Autodesk Fusion 360 part; units mm, degrees
note: some values were not read from the file. Set by a fixed rule: which face or edge a step refers to.
(part 7 of 20)
  spline S38 degree 5 poles (-7.9771, -12.1359) (-7.9772, -12.1359) (-7.9772, -12.136) (-7.9774, -12.1362) (-7.9776, -12.1365) (-7.9779, -12.137) (-7.9782, -12.1375) (-7.9786, -12.1381) (-7.979, -12.1388) (-7.9794, -12.1395) (-7.9799, -12.1403) (-7.9804, -12.1411) (-7.981, -12.1421) (-7.9816, -12.1431) (-7.9823, -12.1441) (-7.9829, -12.1452) (-7.9836, -12.1464) (-7.9844, -12.1477) (-7.9852, -12.149) (-7.986, -12.1504) (-7.9868, -12.1518) (-7.9877, -12.1533) (-7.9886, -12.1549) (-7.9896, -12.1565) (-7.9905, -12.1582) (-7.9915, -12.16) (-7.9926, -12.1618) (-7.9936, -12.1637) (-7.9947, -12.1656) (-7.9958, -12.1676) (-7.997, -12.1696) (-7.9982, -12.1718) (-7.9994, -12.1739) (-8.0006, -12.1762) (-8.0018, -12.1785) (-8.0031, -12.1808) (-8.0044, -12.1832) (-8.0057, -12.1857) (-8.0071, -12.1882) (-8.0084, -12.1908) (-8.0098, -12.1934) (-8.0113, -12.1961) (-8.0127, -12.1988) (-8.0142, -12.2016) (-8.0156, -12.2045) (-8.0171, -12.2074) (-8.0187, -12.2104) (-8.0202, -12.2134) (-8.0218, -12.2164) (-8.0233, -12.2196) (-8.0249, -12.2228) (-8.0265, -12.226) (-8.0282, -12.2293) (-8.0298, -12.2326) (-8.0315, -12.236) (-8.0332, -12.2395) (-8.0349, -12.243) (-8.0366, -12.2465) (-8.0383, -12.2501) (-8.0401, -12.2538) (-8.0419, -12.2575) (-8.0436, -12.2612) (-8.0454, -12.265) (-8.0472, -12.2689) (-8.0491, -12.2728) (-8.0509, -12.2768) (-8.0527, -12.2808) (-8.0546, -12.2848) (-8.0565, -12.289) (-8.0584, -12.2931) (-8.0603, -12.2973) (-8.0622, -12.3016) (-8.0641, -12.3059) (-8.066, -12.3102) (-8.068, -12.3146) (-8.0699, -12.3191) (-8.0719, -12.3236) (-8.0739, -12.3281) (-8.0759, -12.3327) (-8.0779, -12.3374) (-8.0799, -12.3421) (-8.0819, -12.3468) (-8.0839, -12.3516) (-8.0859, -12.3564) (-8.088, -12.3613) (-8.09, -12.3662) (-8.0921, -12.3712) (-8.0941, -12.3762) (-8.0962, -12.3813) (-8.0983, -12.3864) (-8.1004, -12.3915) (-8.1025, -12.3967) (-8.1046, -12.402) (-8.1067, -12.4073) (-8.1088, -12.4126) (-8.1109, -12.418) (-8.113, -12.4234) (-8.1151, -12.4289) (-8.1173, -12.4344) (-8.1194, -12.4399) (-8.1215, -12.4455) (-8.1237, -12.4512) (-8.1258, -12.4568) (-8.128, -12.4626) (-8.1302, -12.4683) (-8.1323, -12.4742) (-8.1345, -12.48) (-8.1366, -12.4859) (-8.1388, -12.4919) (-8.141, -12.4979) (-8.1432, -12.5039) (-8.1453, -12.51) (-8.1475, -12.5161) (-8.1497, -12.5222) (-8.1519, -12.5284) (-8.1541, -12.5347) (-8.1563, -12.5409) (-8.1584, -12.5473) (-8.1606, -12.5536) (-8.1628, -12.56) (-8.165, -12.5665) (-8.1672, -12.5729) (-8.1694, -12.5795) (-8.1716, -12.586) (-8.1738, -12.5926) (-8.176, -12.5993) (-8.1782, -12.606) (-8.1803, -12.6127) (-8.1825, -12.6195) (-8.1847, -12.6263) (-8.1869, -12.6331) (-8.1891, -12.64) (-8.1913, -12.6469) (-8.1935, -12.6539) (-8.1956, -12.6609) (-8.1978, -12.6679) (-8.2, -12.675) (-8.2022, -12.6821) (-8.2044, -12.6893) (-8.2065, -12.6965) (-8.2087, -12.7037) (-8.2109, -12.711) (-8.213, -12.7183) (-8.2152, -12.7256) (-8.2173, -12.733) (-8.2195, -12.7404) (-8.2216, -12.7479) (-8.2238, -12.7554) (-8.2259, -12.7629) (-8.2281, -12.7705) (-8.2302, -12.7781) (-8.2323, -12.7857) (-8.2345, -12.7934) (-8.2366, -12.8011) (-8.2387, -12.8089) (-8.2408, -12.8167) (-8.2429, -12.8245) (-8.245, -12.8324) (-8.2471, -12.8403) (-8.2492, -12.8482) (-8.2513, -12.8562) (-8.2534, -12.8642) (-8.2554, -12.8722) (-8.2575, -12.8803) (-8.2596, -12.8884) (-8.2616, -12.8966) (-8.2637, -12.9048) (-8.2657, -12.913) (-8.2678, -12.9212) (-8.2698, -12.9295) (-8.2718, -12.9379) (-8.2738, -12.9462) (-8.2759, -12.9546) (-8.2779, -12.963) (-8.2799, -12.9715) (-8.2818, -12.98) (-8.2838, -12.9885) (-8.2858, -12.9971) (-8.2878, -13.0057) (-8.2897, -13.0143) (-8.2917, -13.023) (-8.2936, -13.0317) (-8.2956, -13.0404) (-8.2975, -13.0492) (-8.2994, -13.058) (-8.3013, -13.0668) (-8.3032, -13.0757) (-8.3051, -13.0846) (-8.307, -13.0935) (-8.3089, -13.1025) (-8.3107, -13.1115) (-8.3126, -13.1205) (-8.3145, -13.1296) (-8.3163, -13.1386) (-8.3181, -13.1478) (-8.3199, -13.1569) (-8.3218, -13.1661) (-8.3236, -13.1753) (-8.3254, -13.1846) (-8.3271, -13.1939) (-8.3289, -13.2032) (-8.3307, -13.2125) (-8.3324, -13.2219) (-8.3342, -13.2313) (-8.3359, -13.2408) (-8.3376, -13.2503) (-8.3393, -13.2598) (-8.341, -13.2693) (-8.3427, -13.2789) (-8.3444, -13.2885) (-8.3461, -13.2981) (-8.3477, -13.3078) (-8.3494, -13.3174) (-8.351, -13.3272) (-8.3526, -13.3369) (-8.3542, -13.3467) (-8.3558, -13.3565) (-8.3574, -13.3663) (-8.359, -13.3762) (-8.3606, -13.3861) (-8.3621, -13.396) (-8.3637, -13.406) (-8.3652, -13.416) (-8.3667, -13.426) (-8.3682, -13.4361) (-8.3697, -13.4461) (-8.3712, -13.4563) (-8.3726, -13.4664) (-8.3741, -13.4766) (-8.3755, -13.4867) (-8.377, -13.497) (-8.3784, -13.5072) (-8.3798, -13.5175) (-8.3812, -13.5278) (-8.3826, -13.5382) (-8.3839, -13.5485) (-8.3853, -13.5589) (-8.3866, -13.5693) (-8.3879, -13.5798) (-8.3893, -13.5903) (-8.3906, -13.6008) (-8.3916, -13.6092) (-8.3924, -13.6155) (-8.3929, -13.6198) (-8.3931, -13.6219) knots 0 0 0 0 0 0 0.00416667 0.00833333 0.0125 0.01666667 0.02083333 0.025 0.02916667 0.03333333 0.0375 0.04166667 0.04583333 0.05 0.05416667 0.05833333 0.0625 0.06666667 0.07083333 0.075 0.07916667 0.08333333 0.0875 0.09166667 0.09583333 0.1 0.10416667 0.10833333 0.1125 0.11666667 0.12083333 0.125 0.12916667 0.13333333 0.1375 0.14166667 0.14583333 0.15 0.15416667 0.15833333 0.1625 0.16666667 0.17083333 0.175 0.17916667 0.18333333 0.1875 0.19166667 0.19583333 0.2 0.20416667 0.20833333 0.2125 0.21666667 0.22083333 0.225 0.22916667 0.23333333 0.2375 0.24166667 0.24583333 0.25 0.25416667 0.25833333 0.2625 0.26666667 0.27083333 0.275 0.27916667 0.28333333 0.2875 0.29166667 0.29583333 0.3 0.30416667 0.30833333 0.3125 0.31666667 0.32083333 0.325 0.32916667 0.33333333 0.3375 0.34166667 0.34583333 0.35 0.35416667 0.35833333 0.3625 0.36666667 0.37083333 0.375 0.37916667 0.38333333 0.3875 0.39166667 0.39583333 0.4 0.40416667 0.40833333 0.4125 0.41666667 0.42083333 0.425 0.42916667 0.43333333 0.4375 0.44166667 0.44583333 0.45 0.45416667 0.45833333 0.4625 0.46666667 0.47083333 0.475 0.47916667 0.48333333 0.4875 0.49166667 0.49583333 0.5 0.50416667 0.50833333 0.5125 0.51666667 0.52083333 0.525 0.52916667 0.53333333 0.5375 0.54166667 0.54583333 0.55 0.55416667 0.55833333 0.5625 0.56666667 0.57083333 0.575 0.57916667 0.58333333 0.5875 0.59166667 0.59583333 0.6 0.60416667 0.60833333 0.6125 0.61666667 0.62083333 0.625 0.62916667 0.63333333 0.6375 0.64166667 0.64583333 0.65 0.65416667 0.65833333 0.6625 0.66666667 0.67083333 0.675 0.67916667 0.68333333 0.6875 0.69166667 0.69583333 0.7 0.70416667 0.70833333 0.7125 0.71666667 0.72083333 0.725 0.72916667 0.73333333 0.7375 0.74166667 0.74583333 0.75 0.75416667 0.75833333 0.7625 0.76666667 0.77083333 0.775 0.77916667 0.78333333 0.7875 0.79166667 0.79583333 0.8 0.80416667 0.80833333 0.8125 0.81666667 0.82083333 0.825 0.82916667 0.83333333 0.8375 0.84166667 0.84583333 0.85 0.85416667 0.85833333 0.8625 0.86666667 0.87083333 0.875 0.87916667 0.88333333 0.8875 0.89166667 0.89583333 0.9 0.90416667 0.90833333 0.9125 0.91666667 0.92083333 0.925 0.92916667 0.93333333 0.9375 0.94166667 0.94583333 0.95 0.95416667 0.95833333 0.9625 0.96666667 0.97083333 0.975 0.97916667 0.98333333 0.9875 0.99166667 0.99583333 1 1 1 1 1 1
  spline S39 degree 5 poles (-7.6003, -14.0796) (-7.5986, -14.0783) (-7.5952, -14.0758) (-7.5901, -14.0719) (-7.5833, -14.0668) (-7.5749, -14.0604) (-7.5665, -14.0541) (-7.5581, -14.0477) (-7.5497, -14.0413) (-7.5414, -14.035) (-7.5331, -14.0286) (-7.5248, -14.0222) (-7.5166, -14.0159) (-7.5084, -14.0095) (-7.5002, -14.0032) (-7.4921, -13.9968) (-7.484, -13.9905) (-7.4759, -13.9841) (-7.4679, -13.9778) (-7.4599, -13.9714) (-7.4519, -13.9651) (-7.4439, -13.9588) (-7.436, -13.9525) (-7.4281, -13.9461) (-7.4203, -13.9398) (-7.4124, -13.9335) (-7.4046, -13.9272) (-7.3969, -13.9209) (-7.3892, -13.9146) (-7.3815, -13.9083) (-7.3738, -13.902) (-7.3662, -13.8958) (-7.3586, -13.8895) (-7.351, -13.8832) (-7.3435, -13.8769) (-7.336, -13.8707) (-7.3285, -13.8644) (-7.321, -13.8582) (-7.3136, -13.8519) (-7.3063, -13.8457) (-7.2989, -13.8395) (-7.2916, -13.8333) (-7.2843, -13.827) (-7.2771, -13.8208) (-7.2699, -13.8146) (-7.2627, -13.8084) (-7.2555, -13.8023) (-7.2484, -13.7961) (-7.2413, -13.7899) (-7.2343, -13.7837) (-7.2272, -13.7776) (-7.2203, -13.7714) (-7.2133, -13.7653) (-7.2064, -13.7592) (-7.1995, -13.753) (-7.1926, -13.7469) (-7.1858, -13.7408) (-7.179, -13.7347) (-7.1723, -13.7286) (-7.1655, -13.7226) (-7.1588, -13.7165) (-7.1522, -13.7104) (-7.1455, -13.7044) (-7.1389, -13.6983) (-7.1324, -13.6923) (-7.1259, -13.6863) (-7.1194, -13.6803) (-7.1129, -13.6743) (-7.1065, -13.6683) (-7.1001, -13.6623) (-7.0937, -13.6563) (-7.0874, -13.6504) (-7.0811, -13.6444) (-7.0748, -13.6385) (-7.0686, -13.6325) (-7.0624, -13.6266) (-7.0562, -13.6207) (-7.0501, -13.6148) (-7.044, -13.6089) (-7.0379, -13.6031) (-7.0319, -13.5972) (-7.0259, -13.5914) (-7.02, -13.5855) (-7.014, -13.5797) (-7.0081, -13.5739) (-7.0023, -13.5681) (-6.9965, -13.5624) (-6.9907, -13.5566) (-6.9849, -13.5508) (-6.9792, -13.5451) (-6.9735, -13.5394) (-6.9678, -13.5337) (-6.9622, -13.528) (-6.9566, -13.5223) (-6.9511, -13.5166) (-6.9455, -13.511) (-6.94, -13.5053) (-6.9346, -13.4997) (-6.9292, -13.4941) (-6.9238, -13.4885) (-6.9184, -13.4829) (-6.9131, -13.4774) (-6.9078, -13.4718) (-6.9026, -13.4663) (-6.8974, -13.4608) (-6.8922, -13.4553) (-6.8871, -13.4498) (-6.8819, -13.4444) (-6.8769, -13.4389) (-6.8718, -13.4335) (-6.8668, -13.4281) (-6.8618, -13.4227) (-6.8569, -13.4173) (-6.852, -13.412) (-6.8471, -13.4066) (-6.8423, -13.4013) (-6.8375, -13.396) (-6.8327, -13.3907) (-6.828, -13.3855) (-6.8233, -13.3802) (-6.8187, -13.375) (-6.814, -13.3698) (-6.8094, -13.3646) (-6.8049, -13.3595) (-6.8004, -13.3543) (-6.7959, -13.3492) (-6.7914, -13.3441) (-6.787, -13.339) (-6.7826, -13.334) (-6.7783, -13.329) (-6.774, -13.3239) (-6.7697, -13.319) (-6.7655, -13.314) (-6.7613, -13.309) (-6.7571, -13.3041) (-6.753, -13.2992) (-6.7489, -13.2944) (-6.7448, -13.2895) (-6.7408, -13.2847) (-6.7368, -13.2799) (-6.7328, -13.2751) (-6.7289, -13.2703) (-6.725, -13.2656) (-6.7212, -13.2609) (-6.7174, -13.2562) (-6.7136, -13.2516) (-6.7098, -13.2469) (-6.7061, -13.2423) (-6.7025, -13.2378) (-6.6988, -13.2332) (-6.6952, -13.2287) (-6.6917, -13.2242) (-6.6881, -13.2197) (-6.6846, -13.2153) (-6.6812, -13.2109) (-6.6778, -13.2065) (-6.6744, -13.2022) (-6.671, -13.1978) (-6.6677, -13.1935) (-6.6644, -13.1893) (-6.6612, -13.185) (-6.658, -13.1808) (-6.6548, -13.1767) (-6.6517, -13.1725) (-6.6486, -13.1684) (-6.6455, -13.1643) (-6.6425, -13.1603) (-6.6395, -13.1563) (-6.6366, -13.1523) (-6.6337, -13.1483) (-6.6308, -13.1444) (-6.628, -13.1405) (-6.6252, -13.1367) (-6.6224, -13.1328) (-6.6197, -13.1291) (-6.617, -13.1253) (-6.6143, -13.1216) (-6.6117, -13.1179) (-6.6091, -13.1143) (-6.6065, -13.1107) (-6.604, -13.1071) (-6.6016, -13.1036) (-6.5991, -13.1001) (-6.5967, -13.0966) (-6.5944, -13.0932) (-6.592, -13.0898) (-6.5897, -13.0865) (-6.5875, -13.0832) (-6.5853, -13.0799) (-6.5831, -13.0767) (-6.581, -13.0735) (-6.5788, -13.0703) (-6.5768, -13.0672) (-6.5747, -13.0642) (-6.5728, -13.0612) (-6.5708, -13.0582) (-6.5689, -13.0553) (-6.567, -13.0524) (-6.5651, -13.0495) (-6.5633, -13.0467) (-6.5616, -13.044) (-6.5598, -13.0413) (-6.5581, -13.0386) (-6.5565, -13.036) (-6.5549, -13.0334) (-6.5533, -13.0309) (-6.5517, -13.0284) (-6.5502, -13.026) (-6.5488, -13.0236) (-6.5473, -13.0213) (-6.5459, -13.019) (-6.5446, -13.0168) (-6.5433, -13.0146) (-6.542, -13.0125) (-6.5407, -13.0104) (-6.5395, -13.0084) (-6.5384, -13.0064) (-6.5372, -13.0045) (-6.5361, -13.0027) (-6.5351, -13.0009) (-6.5341, -12.9991) (-6.5331, -12.9974) (-6.5321, -12.9958) (-6.5312, -12.9942) (-6.5304, -12.9927) (-6.5295, -12.9913) (-6.5288, -12.9899) (-6.528, -12.9885) (-6.5273, -12.9873) (-6.5266, -12.986) (-6.526, -12.9849) (-6.5254, -12.9838) (-6.5248, -12.9828) (-6.5243, -12.9818) (-6.5238, -12.9809) (-6.5234, -12.9801) (-6.523, -12.9794) (-6.5226, -12.9787) (-6.5223, -12.9781) (-6.522, -12.9775) (-6.5218, -12.977) (-6.5216, -12.9767) (-6.5215, -12.9765) (-6.5214, -12.9764) (-6.5214, -12.9763) knots -1 -1 -1 -1 -1 -1 -0.99583333 -0.99166667 -0.9875 -0.98333333 -0.97916667 -0.975 -0.97083333 -0.96666667 -0.9625 -0.95833333 -0.95416667 -0.95 -0.94583333 -0.94166667 -0.9375 -0.93333333 -0.92916667 -0.925 -0.92083333 -0.91666667 -0.9125 -0.90833333 -0.90416667 -0.9 -0.89583333 -0.89166667 -0.8875 -0.88333333 -0.87916667 -0.875 -0.87083333 -0.86666667 -0.8625 -0.85833333 -0.85416667 -0.85 -0.84583333 -0.84166667 -0.8375 -0.83333333 -0.82916667 -0.825 -0.82083333 -0.81666667 -0.8125 -0.80833333 -0.80416667 -0.8 -0.79583333 -0.79166667 -0.7875 -0.78333333 -0.77916667 -0.775 -0.77083333 -0.76666667 -0.7625 -0.75833333 -0.75416667 -0.75 -0.74583333 -0.74166667 -0.7375 -0.73333333 -0.72916667 -0.725 -0.72083333 -0.71666667 -0.7125 -0.70833333 -0.70416667 -0.7 -0.69583333 -0.69166667 -0.6875 -0.68333333 -0.67916667 -0.675 -0.67083333 -0.66666667 -0.6625 -0.65833333 -0.65416667 -0.65 -0.64583333 -0.64166667 -0.6375 -0.63333333 -0.62916667 -0.625 -0.62083333 -0.61666667 -0.6125 -0.60833333 -0.60416667 -0.6 -0.59583333 -0.59166667 -0.5875 -0.58333333 -0.57916667 -0.575 -0.57083333 -0.56666667 -0.5625 -0.55833333 -0.55416667 -0.55 -0.54583333 -0.54166667 -0.5375 -0.53333333 -0.52916667 -0.525 -0.52083333 -0.51666667 -0.5125 -0.50833333 -0.50416667 -0.5 -0.49583333 -0.49166667 -0.4875 -0.48333333 -0.47916667 -0.475 -0.47083333 -0.46666667 -0.4625 -0.45833333 -0.45416667 -0.45 -0.44583333 -0.44166667 -0.4375 -0.43333333 -0.42916667 -0.425 -0.42083333 -0.41666667 -0.4125 -0.40833333 -0.40416667 -0.4 -0.39583333 -0.39166667 -0.3875 -0.38333333 -0.37916667 -0.375 -0.37083333 -0.36666667 -0.3625 -0.35833333 -0.35416667 -0.35 -0.34583333 -0.34166667 -0.3375 -0.33333333 -0.32916667 -0.325 -0.32083333 -0.31666667 -0.3125 -0.30833333 -0.30416667 -0.3 -0.29583333 -0.29166667 -0.2875 -0.28333333 -0.27916667 -0.275 -0.27083333 -0.26666667 -0.2625 -0.25833333 -0.25416667 -0.25 -0.24583333 -0.24166667 -0.2375 -0.23333333 -0.22916667 -0.225 -0.22083333 -0.21666667 -0.2125 -0.20833333 -0.20416667 -0.2 -0.19583333 -0.19166667 -0.1875 -0.18333333 -0.17916667 -0.175 -0.17083333 -0.16666667 -0.1625 -0.15833333 -0.15416667 -0.15 -0.14583333 -0.14166667 -0.1375 -0.13333333 -0.12916667 -0.125 -0.12083333 -0.11666667 -0.1125 -0.10833333 -0.10416667 -0.1 -0.09583333 -0.09166667 -0.0875 -0.08333333 -0.07916667 -0.075 -0.07083333 -0.06666667 -0.0625 -0.05833333 -0.05416667 -0.05 -0.04583333 -0.04166667 -0.0375 -0.03333333 -0.02916667 -0.025 -0.02083333 -0.01666667 -0.0125 -0.00833333 -0.00416667 0 0 0 0 0 0
  arc A52 (11.0419, 11.5792) -> (10.3616, 12.1917) centre (0, 0) ccw
  line L82 (11.2355, 9.202) -> (11.235, 9.2016)
  spline S40 degree 5 poles (14.4246, 6.9233) (14.4224, 6.9232) (14.4182, 6.9232) (14.4118, 6.9231) (14.4033, 6.9229) (14.3927, 6.9227) (14.3822, 6.9225) (14.3716, 6.9223) (14.3611, 6.9221) (14.3507, 6.9218) (14.3402, 6.9215) (14.3298, 6.9212) (14.3194, 6.9209) (14.309, 6.9206) (14.2987, 6.9203) (14.2883, 6.9199) (14.2781, 6.9195) (14.2678, 6.9192) (14.2576, 6.9188) (14.2474, 6.9183) (14.2372, 6.9179) (14.227, 6.9175) (14.2169, 6.917) (14.2068, 6.9165) (14.1967, 6.916) (14.1867, 6.9155) (14.1767, 6.915) (14.1667, 6.9145) (14.1568, 6.9139) (14.1468, 6.9134) (14.1369, 6.9128) (14.1271, 6.9122) (14.1172, 6.9116) (14.1074, 6.9109) (14.0976, 6.9103) (14.0879, 6.9097) (14.0782, 6.909) (14.0685, 6.9083) (14.0588, 6.9076) (14.0492, 6.9069) (14.0396, 6.9062) (14.03, 6.9055) (14.0205, 6.9047) (14.011, 6.9039) (14.0015, 6.9032) (13.992, 6.9024) (13.9826, 6.9016) (13.9732, 6.9008) (13.9639, 6.8999) (13.9545, 6.8991) (13.9452, 6.8982) (13.936, 6.8974) (13.9267, 6.8965) (13.9175, 6.8956) (13.9083, 6.8947) (13.8992, 6.8938) (13.8901, 6.8929) (13.881, 6.8919) (13.872, 6.891) (13.8629, 6.89) (13.854, 6.889) (13.845, 6.888) (13.8361, 6.887) (13.8272, 6.886) (13.8184, 6.885) (13.8095, 6.884) (13.8007, 6.8829) (13.792, 6.8818) (13.7833, 6.8808) (13.7746, 6.8797) (13.7659, 6.8786) (13.7573, 6.8775) (13.7487, 6.8764) (13.7401, 6.8753) (13.7316, 6.8741) (13.7231, 6.873) (13.7147, 6.8718) (13.7063, 6.8707) (13.6979, 6.8695) (13.6895, 6.8683) (13.6812, 6.8671) (13.6729, 6.8659) (13.6647, 6.8647) (13.6564, 6.8635) (13.6483, 6.8623) (13.6401, 6.861) (13.632, 6.8598) (13.6239, 6.8585) (13.6159, 6.8572) (13.6079, 6.856) (13.5999, 6.8547) (13.592, 6.8534) (13.5841, 6.8521) (13.5762, 6.8508) (13.5684, 6.8494) (13.5606, 6.8481) (13.5528, 6.8468) (13.5451, 6.8454) (13.5375, 6.8441) (13.5298, 6.8427) (13.5222, 6.8414) (13.5146, 6.84) (13.5071, 6.8386) (13.4996, 6.8372) (13.4922, 6.8358) (13.4847, 6.8344) (13.4773, 6.833) (13.47, 6.8316) (13.4627, 6.8302) (13.4554, 6.8288) (13.4482, 6.8273) (13.441, 6.8259) (13.4339, 6.8244) (13.4267, 6.823) (13.4197, 6.8215) (13.4126, 6.8201) (13.4056, 6.8186) (13.3987, 6.8171) (13.3918, 6.8157) (13.3849, 6.8142) (13.378, 6.8127) (13.3712, 6.8112) (13.3645, 6.8097) (13.3578, 6.8082) (13.3511, 6.8067) (13.3445, 6.8052) (13.3379, 6.8037) (13.3313, 6.8022) (13.3248, 6.8007) (13.3183, 6.7992) (13.3119, 6.7976) (13.3055, 6.7961) (13.2991, 6.7946) (13.2928, 6.7931) (13.2866, 6.7915) (13.2804, 6.79) (13.2742, 6.7885) (13.268, 6.7869) (13.2619, 6.7854) (13.2559, 6.7839) (13.2499, 6.7823) (13.2439, 6.7808) (13.238, 6.7792) (13.2321, 6.7777) (13.2263, 6.7761) (13.2205, 6.7746) (13.2147, 6.7731) (13.209, 6.7715) (13.2034, 6.77) (13.1978, 6.7684) (13.1922, 6.7669) (13.1867, 6.7653) (13.1812, 6.7638) (13.1758, 6.7623) (13.1704, 6.7607) (13.165, 6.7592) (13.1597, 6.7577) (13.1545, 6.7561) (13.1493, 6.7546) (13.1441, 6.7531) (13.139, 6.7516) (13.1339, 6.75) (13.1289, 6.7485) (13.124, 6.747) (13.119, 6.7455) (13.1142, 6.744) (13.1093, 6.7425) (13.1046, 6.741) (13.0998, 6.7395) (13.0951, 6.738) (13.0905, 6.7366) (13.0859, 6.7351) (13.0814, 6.7336) (13.0769, 6.7321) (13.0725, 6.7307) (13.0681, 6.7292) (13.0638, 6.7278) (13.0595, 6.7264) (13.0552, 6.7249) (13.0511, 6.7235) (13.0469, 6.7221) (13.0429, 6.7207) (13.0388, 6.7193) (13.0349, 6.7179) (13.0309, 6.7165) (13.0271, 6.7152) (13.0232, 6.7138) (13.0195, 6.7125) (13.0158, 6.7111) (13.0121, 6.7098) (13.0085, 6.7085) (13.005, 6.7072) (13.0015, 6.7059) (12.998, 6.7046) (12.9946, 6.7033) (12.9913, 6.7021) (12.988, 6.7008) (12.9848, 6.6996) (12.9816, 6.6984) (12.9785, 6.6972) (12.9755, 6.696) (12.9725, 6.6948) (12.9695, 6.6937) (12.9667, 6.6925) (12.9638, 6.6914) (12.9611, 6.6903) (12.9584, 6.6892) (12.9557, 6.6881) (12.9531, 6.6871) (12.9506, 6.686) (12.9482, 6.685) (12.9457, 6.684) (12.9434, 6.683) (12.9411, 6.6821) (12.9389, 6.6811) (12.9367, 6.6802) (12.9346, 6.6793) (12.9326, 6.6784) (12.9306, 6.6775) (12.9287, 6.6767) (12.9269, 6.6759) (12.9251, 6.6751) (12.9234, 6.6743) (12.9217, 6.6736) (12.9201, 6.6729) (12.9186, 6.6722) (12.9171, 6.6715) (12.9157, 6.6709) (12.9144, 6.6703) (12.9132, 6.6697) (12.912, 6.6691) (12.9108, 6.6686) (12.9098, 6.6681) (12.9088, 6.6676) (12.9079, 6.6672) (12.9071, 6.6668) (12.9063, 6.6664) (12.9056, 6.6661) (12.905, 6.6658) (12.9044, 6.6655) (12.9039, 6.6652) (12.9036, 6.6651) (12.9034, 6.665) (12.9033, 6.6649) (12.9032, 6.6649) knots -1 -1 -1 -1 -1 -1 -0.99583333 -0.99166667 -0.9875 -0.98333333 -0.97916667 -0.975 -0.97083333 -0.96666667 -0.9625 -0.95833333 -0.95416667 -0.95 -0.94583333 -0.94166667 -0.9375 -0.93333333 -0.92916667 -0.925 -0.92083333 -0.91666667 -0.9125 -0.90833333 -0.90416667 -0.9 -0.89583333 -0.89166667 -0.8875 -0.88333333 -0.87916667 -0.875 -0.87083333 -0.86666667 -0.8625 -0.85833333 -0.85416667 -0.85 -0.84583333 -0.84166667 -0.8375 -0.83333333 -0.82916667 -0.825 -0.82083333 -0.81666667 -0.8125 -0.80833333 -0.80416667 -0.8 -0.79583333 -0.79166667 -0.7875 -0.78333333 -0.77916667 -0.775 -0.77083333 -0.76666667 -0.7625 -0.75833333 -0.75416667 -0.75 -0.74583333 -0.74166667 -0.7375 -0.73333333 -0.72916667 -0.725 -0.72083333 -0.71666667 -0.7125 -0.70833333 -0.70416667 -0.7 -0.69583333 -0.69166667 -0.6875 -0.68333333 -0.67916667 -0.675 -0.67083333 -0.66666667 -0.6625 -0.65833333 -0.65416667 -0.65 -0.64583333 -0.64166667 -0.6375 -0.63333333 -0.62916667 -0.625 -0.62083333 -0.61666667 -0.6125 -0.60833333 -0.60416667 -0.6 -0.59583333 -0.59166667 -0.5875 -0.58333333 -0.57916667 -0.575 -0.57083333 -0.56666667 -0.5625 -0.55833333 -0.55416667 -0.55 -0.54583333 -0.54166667 -0.5375 -0.53333333 -0.52916667 -0.525 -0.52083333 -0.51666667 -0.5125 -0.50833333 -0.50416667 -0.5 -0.49583333 -0.49166667 -0.4875 -0.48333333 -0.47916667 -0.475 -0.47083333 -0.46666667 -0.4625 -0.45833333 -0.45416667 -0.45 -0.44583333 -0.44166667 -0.4375 -0.43333333 -0.42916667 -0.425 -0.42083333 -0.41666667 -0.4125 -0.40833333 -0.40416667 -0.4 -0.39583333 -0.39166667 -0.3875 -0.38333333 -0.37916667 -0.375 -0.37083333 -0.36666667 -0.3625 -0.35833333 -0.35416667 -0.35 -0.34583333 -0.34166667 -0.3375 -0.33333333 -0.32916667 -0.325 -0.32083333 -0.31666667 -0.3125 -0.30833333 -0.30416667 -0.3 -0.29583333 -0.29166667 -0.2875 -0.28333333 -0.27916667 -0.275 -0.27083333 -0.26666667 -0.2625 -0.25833333 -0.25416667 -0.25 -0.24583333 -0.24166667 -0.2375 -0.23333333 -0.22916667 -0.225 -0.22083333 -0.21666667 -0.2125 -0.20833333 -0.20416667 -0.2 -0.19583333 -0.19166667 -0.1875 -0.18333333 -0.17916667 -0.175 -0.17083333 -0.16666667 -0.1625 -0.15833333 -0.15416667 -0.15 -0.14583333 -0.14166667 -0.1375 -0.13333333 -0.12916667 -0.125 -0.12083333 -0.11666667 -0.1125 -0.10833333 -0.10416667 -0.1 -0.09583333 -0.09166667 -0.0875 -0.08333333 -0.07916667 -0.075 -0.07083333 -0.06666667 -0.0625 -0.05833333 -0.05416667 -0.05 -0.04583333 -0.04166667 -0.0375 -0.03333333 -0.02916667 -0.025 -0.02083333 -0.01666667 -0.0125 -0.00833333 -0.00416667 0 0 0 0 0 0
  line L83 (-3.4851, 13.301) -> (-3.6808, 14.048)
  spline S41 degree 5 poles (10.3616, 12.1917) (10.3596, 12.1908) (10.3558, 12.189) (10.35, 12.1863) (10.3423, 12.1828) (10.3327, 12.1783) (10.3231, 12.1738) (10.3136, 12.1693) (10.3041, 12.1648) (10.2946, 12.1603) (10.2852, 12.1558) (10.2758, 12.1513) (10.2664, 12.1468) (10.2571, 12.1423) (10.2478, 12.1378) (10.2385, 12.1332) (10.2292, 12.1287) (10.22, 12.1242) (10.2108, 12.1197) (10.2017, 12.1151) (10.1925, 12.1106) (10.1834, 12.1061) (10.1744, 12.1015) (10.1654, 12.097) (10.1564, 12.0924) (10.1474, 12.0879) (10.1385, 12.0834) (10.1296, 12.0788) (10.1207, 12.0743) (10.1119, 12.0697) (10.1031, 12.0651) (10.0943, 12.0606) (10.0855, 12.056) (10.0768, 12.0515) (10.0682, 12.0469) (10.0595, 12.0423) (10.0509, 12.0378) (10.0423, 12.0332) (10.0338, 12.0287) (10.0253, 12.0241) (10.0168, 12.0195) (10.0084, 12.015) (9.9999, 12.0104) (9.9916, 12.0058) (9.9832, 12.0013) (9.9749, 11.9967) (9.9666, 11.9921) (9.9584, 11.9876) (9.9502, 11.983) (9.942, 11.9785) (9.9338, 11.9739) (9.9257, 11.9693) (9.9176, 11.9648) (9.9096, 11.9602) (9.9016, 11.9557) (9.8936, 11.9511) (9.8857, 11.9465) (9.8777, 11.942) (9.8699, 11.9374) (9.862, 11.9329) (9.8542, 11.9283) (9.8464, 11.9238) (9.8387, 11.9193) (9.831, 11.9147) (9.8233, 11.9102) (9.8157, 11.9056) (9.8081, 11.9011) (9.8005, 11.8966) (9.793, 11.8921) (9.7855, 11.8875) (9.778, 11.883) (9.7706, 11.8785) (9.7632, 11.874) (9.7558, 11.8695) (9.7485, 11.865) (9.7412, 11.8605) (9.7339, 11.856) (9.7267, 11.8515) (9.7195, 11.847) (9.7124, 11.8425) (9.7053, 11.8381) (9.6982, 11.8336) (9.6912, 11.8291) (9.6841, 11.8247) (9.6772, 11.8202) (9.6702, 11.8158) (9.6633, 11.8113) (9.6565, 11.8069) (9.6496, 11.8025) (9.6428, 11.798) (9.6361, 11.7936) (9.6294, 11.7892) (9.6227, 11.7848) (9.616, 11.7804) (9.6094, 11.776) (9.6028, 11.7717) (9.5963, 11.7673) (9.5898, 11.7629) (9.5833, 11.7586) (9.5769, 11.7542) (9.5705, 11.7499) (9.5642, 11.7455) (9.5578, 11.7412) (9.5516, 11.7369) (9.5453, 11.7326) (9.5391, 11.7283) (9.5329, 11.724) (9.5268, 11.7197) (9.5207, 11.7155) (9.5146, 11.7112) (9.5086, 11.707) (9.5026, 11.7027) (9.4967, 11.6985) (9.4908, 11.6943) (9.4849, 11.6901) (9.4791, 11.6859) (9.4733, 11.6817) (9.4675, 11.6775) (9.4618, 11.6733) (9.4561, 11.6692) (9.4505, 11.6651) (9.4449, 11.6609) (9.4393, 11.6568) (9.4338, 11.6527) (9.4283, 11.6486) (9.4228, 11.6446) (9.4174, 11.6405) (9.412, 11.6365) (9.4067, 11.6324) (9.4014, 11.6284) (9.3962, 11.6244) (9.3909, 11.6204) (9.3858, 11.6164) (9.3806, 11.6125) (9.3755, 11.6085) (9.3705, 11.6046) (9.3654, 11.6007) (9.3605, 11.5968) (9.3555, 11.5929) (9.3506, 11.589) (9.3457, 11.5852) (9.3409, 11.5813) (9.3361, 11.5775) (9.3314, 11.5737) (9.3267, 11.5699) (9.322, 11.5662) (9.3174, 11.5624) (9.3128, 11.5587) (9.3083, 11.555) (9.3038, 11.5513) (9.2993, 11.5476) (9.2949, 11.544) (9.2905, 11.5403) (9.2862, 11.5367) (9.2819, 11.5331) (9.2776, 11.5295) (9.2734, 11.526) (9.2692, 11.5224) (9.2651, 11.5189) (9.261, 11.5154) (9.257, 11.512) (9.253, 11.5085) (9.249, 11.5051) (9.2451, 11.5017) (9.2412, 11.4983) (9.2373, 11.495) (9.2335, 11.4916) (9.2298, 11.4883) (9.2261, 11.485) (9.2224, 11.4818) (9.2188, 11.4785) (9.2152, 11.4753) (9.2116, 11.4721) (9.2081, 11.469) (9.2047, 11.4658) (9.2013, 11.4627) (9.1979, 11.4597) (9.1946, 11.4566) (9.1913, 11.4536) (9.188, 11.4506) (9.1848, 11.4476) (9.1817, 11.4447) (9.1786, 11.4418) (9.1755, 11.4389) (9.1725, 11.436) (9.1695, 11.4332) (9.1666, 11.4304) (9.1637, 11.4276) (9.1608, 11.4249) (9.158, 11.4222) (9.1553, 11.4195) (9.1526, 11.4169) (9.1499, 11.4143) (9.1473, 11.4117) (9.1447, 11.4092) (9.1422, 11.4067) (9.1397, 11.4042) (9.1372, 11.4018) (9.1348, 11.3994) (9.1325, 11.397) (9.1302, 11.3947) (9.1279, 11.3924) (9.1257, 11.3902) (9.1235, 11.388) (9.1214, 11.3858) (9.1194, 11.3836) (9.1173, 11.3815) (9.1153, 11.3795) (9.1134, 11.3775) (9.1115, 11.3755) (9.1097, 11.3735) (9.1079, 11.3717) (9.1062, 11.3698) (9.1045, 11.368) (9.1028, 11.3662) (9.1012, 11.3645) (9.0997, 11.3628) (9.0982, 11.3612) (9.0967, 11.3596) (9.0953, 11.3581) (9.0939, 11.3566) (9.0926, 11.3551) (9.0914, 11.3537) (9.0902, 11.3524) (9.089, 11.3511) (9.0879, 11.3498) (9.0868, 11.3486) (9.0858, 11.3475) (9.0849, 11.3464) (9.084, 11.3453) (9.0831, 11.3443) (9.0823, 11.3434) (9.0815, 11.3425) (9.0808, 11.3417) (9.0802, 11.3409) (9.0796, 11.3402) (9.079, 11.3395) (9.0785, 11.3389) (9.0781, 11.3384) (9.0777, 11.3379) (9.0773, 11.3375) (9.0771, 11.3372) (9.0769, 11.337) (9.0769, 11.3369) (9.0768, 11.3369) knots -1 -1 -1 -1 -1 -1 -0.99583333 -0.99166667 -0.9875 -0.98333333 -0.97916667 -0.975 -0.97083333 -0.96666667 -0.9625 -0.95833333 -0.95416667 -0.95 -0.94583333 -0.94166667 -0.9375 -0.93333333 -0.92916667 -0.925 -0.92083333 -0.91666667 -0.9125 -0.90833333 -0.90416667 -0.9 -0.89583333 -0.89166667 -0.8875 -0.88333333 -0.87916667 -0.875 -0.87083333 -0.86666667 -0.8625 -0.85833333 -0.85416667 -0.85 -0.84583333 -0.84166667 -0.8375 -0.83333333 -0.82916667 -0.825 -0.82083333 -0.81666667 -0.8125 -0.80833333 -0.80416667 -0.8 -0.79583333 -0.79166667 -0.7875 -0.78333333 -0.77916667 -0.775 -0.77083333 -0.76666667 -0.7625 -0.75833333 -0.75416667 -0.75 -0.74583333 -0.74166667 -0.7375 -0.73333333 -0.72916667 -0.725 -0.72083333 -0.71666667 -0.7125 -0.70833333 -0.70416667 -0.7 -0.69583333 -0.69166667 -0.6875 -0.68333333 -0.67916667 -0.675 -0.67083333 -0.66666667 -0.6625 -0.65833333 -0.65416667 -0.65 -0.64583333 -0.64166667 -0.6375 -0.63333333 -0.62916667 -0.625 -0.62083333 -0.61666667 -0.6125 -0.60833333 -0.60416667 -0.6 -0.59583333 -0.59166667 -0.5875 -0.58333333 -0.57916667 -0.575 -0.57083333 -0.56666667 -0.5625 -0.55833333 -0.55416667 -0.55 -0.54583333 -0.54166667 -0.5375 -0.53333333 -0.52916667 -0.525 -0.52083333 -0.51666667 -0.5125 -0.50833333 -0.50416667 -0.5 -0.49583333 -0.49166667 -0.4875 -0.48333333 -0.47916667 -0.475 -0.47083333 -0.46666667 -0.4625 -0.45833333 -0.45416667 -0.45 -0.44583333 -0.44166667 -0.4375 -0.43333333 -0.42916667 -0.425 -0.42083333 -0.41666667 -0.4125 -0.40833333 -0.40416667 -0.4 -0.39583333 -0.39166667 -0.3875 -0.38333333 -0.37916667 -0.375 -0.37083333 -0.36666667 -0.3625 -0.35833333 -0.35416667 -0.35 -0.34583333 -0.34166667 -0.3375 -0.33333333 -0.32916667 -0.325 -0.32083333 -0.31666667 -0.3125 -0.30833333 -0.30416667 -0.3 -0.29583333 -0.29166667 -0.2875 -0.28333333 -0.27916667 -0.275 -0.27083333 -0.26666667 -0.2625 -0.25833333 -0.25416667 -0.25 -0.24583333 -0.24166667 -0.2375 -0.23333333 -0.22916667 -0.225 -0.22083333 -0.21666667 -0.2125 -0.20833333 -0.20416667 -0.2 -0.19583333 -0.19166667 -0.1875 -0.18333333 -0.17916667 -0.175 -0.17083333 -0.16666667 -0.1625 -0.15833333 -0.15416667 -0.15 -0.14583333 -0.14166667 -0.1375 -0.13333333 -0.12916667 -0.125 -0.12083333 -0.11666667 -0.1125 -0.10833333 -0.10416667 -0.1 -0.09583333 -0.09166667 -0.0875 -0.08333333 -0.07916667 -0.075 -0.07083333 -0.06666667 -0.0625 -0.05833333 -0.05416667 -0.05 -0.04583333 -0.04166667 -0.0375 -0.03333333 -0.02916667 -0.025 -0.02083333 -0.01666667 -0.0125 -0.00833333 -0.00416667 0 0 0 0 0 0
  line L84 (11.235, 9.2016) -> (10.6376, 8.7123)
  line L85 (-2.3513, 14.3306) -> (-2.2262, 13.5686)
  spline S42 degree 5 poles (-0.6796, 14.5069) (-0.6796, 14.507) (-0.6797, 14.5072) (-0.6797, 14.5074) (-0.6797, 14.5078) (-0.6797, 14.5083) (-0.6798, 14.5089) (-0.6798, 14.5096) (-0.6799, 14.5104) (-0.6799, 14.5112) (-0.68, 14.5122) (-0.6801, 14.5132) (-0.6802, 14.5143) (-0.6803, 14.5154) (-0.6804, 14.5167) (-0.6805, 14.518) (-0.6806, 14.5193) (-0.6807, 14.5208) (-0.6809, 14.5223) (-0.681, 14.5239) (-0.6812, 14.5256) (-0.6814, 14.5273) (-0.6815, 14.5291) (-0.6817, 14.531) (-0.6819, 14.5329) (-0.6822, 14.5349) (-0.6824, 14.537) (-0.6826, 14.5392) (-0.6829, 14.5414) (-0.6832, 14.5436) (-0.6834, 14.546) (-0.6837, 14.5484) (-0.684, 14.5508) (-0.6844, 14.5533) (-0.6847, 14.5559) (-0.685, 14.5586) (-0.6854, 14.5613) (-0.6858, 14.5641) (-0.6862, 14.5669) (-0.6866, 14.5698) (-0.687, 14.5727) (-0.6874, 14.5757) (-0.6879, 14.5788) (-0.6883, 14.5819) (-0.6888, 14.5851) (-0.6893, 14.5883) (-0.6898, 14.5916) (-0.6904, 14.595) (-0.6909, 14.5984) (-0.6915, 14.6018) (-0.6921, 14.6054) (-0.6926, 14.6089) (-0.6933, 14.6125) (-0.6939, 14.6162) (-0.6945, 14.6199) (-0.6952, 14.6237) (-0.6959, 14.6275) (-0.6966, 14.6314) (-0.6973, 14.6354) (-0.698, 14.6394) (-0.6988, 14.6434) (-0.6995, 14.6475) (-0.7003, 14.6516) (-0.7011, 14.6558) (-0.702, 14.66) (-0.7028, 14.6643) (-0.7037, 14.6686) (-0.7045, 14.673) (-0.7054, 14.6774) (-0.7064, 14.6819) (-0.7073, 14.6864) (-0.7082, 14.691) (-0.7092, 14.6956) (-0.7102, 14.7003) (-0.7112, 14.705) (-0.7123, 14.7097) (-0.7133, 14.7145) (-0.7144, 14.7194) (-0.7155, 14.7243) (-0.7166, 14.7292) (-0.7177, 14.7342) (-0.7189, 14.7392) (-0.7201, 14.7442) (-0.7213, 14.7493) (-0.7225, 14.7545) (-0.7237, 14.7597) (-0.725, 14.7649) (-0.7263, 14.7702) (-0.7276, 14.7755) (-0.7289, 14.7808) (-0.7302, 14.7862) (-0.7316, 14.7917) (-0.733, 14.7971) (-0.7344, 14.8027) (-0.7358, 14.8082) (-0.7372, 14.8138) (-0.7387, 14.8194) (-0.7402, 14.8251) (-0.7417, 14.8308) (-0.7433, 14.8366) (-0.7448, 14.8424) (-0.7464, 14.8482) (-0.748, 14.854) (-0.7496, 14.86) (-0.7513, 14.8659) (-0.7529, 14.8719) (-0.7546, 14.8779) (-0.7564, 14.8839) (-0.7581, 14.89) (-0.7599, 14.8961) (-0.7616, 14.9023) (-0.7634, 14.9085) (-0.7653, 14.9147) (-0.7671, 14.921) (-0.769, 14.9273) (-0.7709, 14.9336) (-0.7728, 14.94) (-0.7748, 14.9464) (-0.7767, 14.9528) (-0.7787, 14.9593) (-0.7807, 14.9658) (-0.7828, 14.9723) (-0.7848, 14.9789) (-0.7869, 14.9855) (-0.789, 14.9921) (-0.7912, 14.9987) (-0.7933, 15.0054) (-0.7955, 15.0122) (-0.7977, 15.0189) (-0.8, 15.0257) (-0.8022, 15.0325) (-0.8045, 15.0394) (-0.8068, 15.0463) (-0.8091, 15.0532) (-0.8115, 15.0601) (-0.8138, 15.0671) (-0.8162, 15.0741) (-0.8187, 15.0812) (-0.8211, 15.0882) (-0.8236, 15.0953) (-0.8261, 15.1025) (-0.8286, 15.1096) (-0.8311, 15.1168) (-0.8337, 15.124) (-0.8363, 15.1313) (-0.8389, 15.1385) (-0.8416, 15.1458) (-0.8442, 15.1531) (-0.8469, 15.1605) (-0.8497, 15.1679) (-0.8524, 15.1753) (-0.8552, 15.1827) (-0.858, 15.1902) (-0.8608, 15.1977) (-0.8636, 15.2052) (-0.8665, 15.2127) (-0.8694, 15.2203) (-0.8723, 15.2279) (-0.8753, 15.2355) (-0.8782, 15.2432) (-0.8812, 15.2509) (-0.8843, 15.2586) (-0.8873, 15.2663) (-0.8904, 15.274) (-0.8935, 15.2818) (-0.8966, 15.2896) (-0.8998, 15.2974) (-0.9029, 15.3053) (-0.9061, 15.3132) (-0.9094, 15.3211) (-0.9126, 15.329) (-0.9159, 15.3369) (-0.9192, 15.3449) (-0.9225, 15.3529) (-0.9259, 15.3609) (-0.9293, 15.369) (-0.9327, 15.377) (-0.9361, 15.3851) (-0.9396, 15.3932) (-0.9431, 15.4014) (-0.9466, 15.4095) (-0.9501, 15.4177) (-0.9537, 15.4259) (-0.9573, 15.4341) (-0.9609, 15.4424) (-0.9646, 15.4507) (-0.9682, 15.459) (-0.9719, 15.4673) (-0.9757, 15.4756) (-0.9794, 15.484) (-0.9832, 15.4923) (-0.987, 15.5007) (-0.9908, 15.5091) (-0.9947, 15.5176) (-0.9986, 15.526) (-1.0025, 15.5345) (-1.0064, 15.543) (-1.0104, 15.5515) (-1.0144, 15.5601) (-1.0184, 15.5686) (-1.0224, 15.5772) (-1.0265, 15.5858) (-1.0306, 15.5944) (-1.0347, 15.6031) (-1.0389, 15.6117) (-1.043, 15.6204) (-1.0472, 15.6291) (-1.0515, 15.6378) (-1.0557, 15.6466) (-1.06, 15.6553) (-1.0643, 15.6641) (-1.0687, 15.6729) (-1.073, 15.6817) (-1.0774, 15.6905) (-1.0818, 15.6993) (-1.0863, 15.7082) (-1.0907, 15.7171) (-1.0952, 15.726) (-1.0998, 15.7349) (-1.1043, 15.7438) (-1.1089, 15.7528) (-1.1135, 15.7617) (-1.1182, 15.7707) (-1.1228, 15.7797) (-1.1275, 15.7887) (-1.1322, 15.7977) (-1.137, 15.8068) (-1.1417, 15.8159) (-1.1465, 15.8249) (-1.1514, 15.834) (-1.1562, 15.8431) (-1.1611, 15.8523) (-1.166, 15.8614) (-1.1709, 15.8706) (-1.1759, 15.8797) (-1.1809, 15.8889) (-1.1859, 15.8981) (-1.1909, 15.9074) (-1.196, 15.9166) (-1.2011, 15.9258) (-1.2062, 15.9351) (-1.2104, 15.9425) (-1.2135, 15.9481) (-1.2155, 15.9518) (-1.2166, 15.9537) knots 0 0 0 0 0 0 0.00416667 0.00833333 0.0125 0.01666667 0.02083333 0.025 0.02916667 0.03333333 0.0375 0.04166667 0.04583333 0.05 0.05416667 0.05833333 0.0625 0.06666667 0.07083333 0.075 0.07916667 0.08333333 0.0875 0.09166667 0.09583333 0.1 0.10416667 0.10833333 0.1125 0.11666667 0.12083333 0.125 0.12916667 0.13333333 0.1375 0.14166667 0.14583333 0.15 0.15416667 0.15833333 0.1625 0.16666667 0.17083333 0.175 0.17916667 0.18333333 0.1875 0.19166667 0.19583333 0.2 0.20416667 0.20833333 0.2125 0.21666667 0.22083333 0.225 0.22916667 0.23333333 0.2375 0.24166667 0.24583333 0.25 0.25416667 0.25833333 0.2625 0.26666667 0.27083333 0.275 0.27916667 0.28333333 0.2875 0.29166667 0.29583333 0.3 0.30416667 0.30833333 0.3125 0.31666667 0.32083333 0.325 0.32916667 0.33333333 0.3375 0.34166667 0.34583333 0.35 0.35416667 0.35833333 0.3625 0.36666667 0.37083333 0.375 0.37916667 0.38333333 0.3875 0.39166667 0.39583333 0.4 0.40416667 0.40833333 0.4125 0.41666667 0.42083333 0.425 0.42916667 0.43333333 0.4375 0.44166667 0.44583333 0.45 0.45416667 0.45833333 0.4625 0.46666667 0.47083333 0.475 0.47916667 0.48333333 0.4875 0.49166667 0.49583333 0.5 0.50416667 0.50833333 0.5125 0.51666667 0.52083333 0.525 0.52916667 0.53333333 0.5375 0.54166667 0.54583333 0.55 0.55416667 0.55833333 0.5625 0.56666667 0.57083333 0.575 0.57916667 0.58333333 0.5875 0.59166667 0.59583333 0.6 0.60416667 0.60833333 0.6125 0.61666667 0.62083333 0.625 0.62916667 0.63333333 0.6375 0.64166667 0.64583333 0.65 0.65416667 0.65833333 0.6625 0.66666667 0.67083333 0.675 0.67916667 0.68333333 0.6875 0.69166667 0.69583333 0.7 0.70416667 0.70833333 0.7125 0.71666667 0.72083333 0.725 0.72916667 0.73333333 0.7375 0.74166667 0.74583333 0.75 0.75416667 0.75833333 0.7625 0.76666667 0.77083333 0.775 0.77916667 0.78333333 0.7875 0.79166667 0.79583333 0.8 0.80416667 0.80833333 0.8125 0.81666667 0.82083333 0.825 0.82916667 0.83333333 0.8375 0.84166667 0.84583333 0.85 0.85416667 0.85833333 0.8625 0.86666667 0.87083333 0.875 0.87916667 0.88333333 0.8875 0.89166667 0.89583333 0.9 0.90416667 0.90833333 0.9125 0.91666667 0.92083333 0.925 0.92916667 0.93333333 0.9375 0.94166667 0.94583333 0.95 0.95416667 0.95833333 0.9625 0.96666667 0.97083333 0.975 0.97916667 0.98333333 0.9875 0.99166667 0.99583333 1 1 1 1 1 1
  spline S43 degree 5 poles (-10.3616, -12.1917) (-10.3596, -12.1908) (-10.3558, -12.189) (-10.35, -12.1863) (-10.3423, -12.1828) (-10.3327, -12.1783) (-10.3231, -12.1738) (-10.3136, -12.1693) (-10.3041, -12.1648) (-10.2946, -12.1603) (-10.2852, -12.1558) (-10.2758, -12.1513) (-10.2664, -12.1468) (-10.2571, -12.1423) (-10.2478, -12.1378) (-10.2385, -12.1332) (-10.2292, -12.1287) (-10.22, -12.1242) (-10.2108, -12.1197) (-10.2017, -12.1151) (-10.1925, -12.1106) (-10.1834, -12.1061) (-10.1744, -12.1015) (-10.1654, -12.097) (-10.1564, -12.0924) (-10.1474, -12.0879) (-10.1385, -12.0834) (-10.1296, -12.0788) (-10.1207, -12.0743) (-10.1119, -12.0697) (-10.1031, -12.0651) (-10.0943, -12.0606) (-10.0855, -12.056) (-10.0768, -12.0515) (-10.0682, -12.0469) (-10.0595, -12.0423) (-10.0509, -12.0378) (-10.0423, -12.0332) (-10.0338, -12.0287) (-10.0253, -12.0241) (-10.0168, -12.0195) (-10.0084, -12.015) (-9.9999, -12.0104) (-9.9916, -12.0058) (-9.9832, -12.0013) (-9.9749, -11.9967) (-9.9666, -11.9921) (-9.9584, -11.9876) (-9.9502, -11.983) (-9.942, -11.9785) (-9.9338, -11.9739) (-9.9257, -11.9693) (-9.9176, -11.9648) (-9.9096, -11.9602) (-9.9016, -11.9557) (-9.8936, -11.9511) (-9.8857, -11.9465) (-9.8777, -11.942) (-9.8699, -11.9374) (-9.862, -11.9329) (-9.8542, -11.9283) (-9.8464, -11.9238) (-9.8387, -11.9193) (-9.831, -11.9147) (-9.8233, -11.9102) (-9.8157, -11.9056) (-9.8081, -11.9011) (-9.8005, -11.8966) (-9.793, -11.8921) (-9.7855, -11.8875) (-9.778, -11.883) (-9.7706, -11.8785) (-9.7632, -11.874) (-9.7558, -11.8695) (-9.7485, -11.865) (-9.7412, -11.8605) (-9.7339, -11.856) (-9.7267, -11.8515) (-9.7195, -11.847) (-9.7124, -11.8425) (-9.7053, -11.8381) (-9.6982, -11.8336) (-9.6912, -11.8291) (-9.6841, -11.8247) (-9.6772, -11.8202) (-9.6702, -11.8158) (-9.6633, -11.8113) (-9.6565, -11.8069) (-9.6496, -11.8025) (-9.6428, -11.798) (-9.6361, -11.7936) (-9.6294, -11.7892) (-9.6227, -11.7848) (-9.616, -11.7804) (-9.6094, -11.776) (-9.6028, -11.7717) (-9.5963, -11.7673) (-9.5898, -11.7629) (-9.5833, -11.7586) (-9.5769, -11.7542) (-9.5705, -11.7499) (-9.5642, -11.7455) (-9.5578, -11.7412) (-9.5516, -11.7369) (-9.5453, -11.7326) (-9.5391, -11.7283) (-9.5329, -11.724) (-9.5268, -11.7197) (-9.5207, -11.7155) (-9.5146, -11.7112) (-9.5086, -11.707) (-9.5026, -11.7027) (-9.4967, -11.6985) (-9.4908, -11.6943) (-9.4849, -11.6901) (-9.4791, -11.6859) (-9.4733, -11.6817) (-9.4675, -11.6775) (-9.4618, -11.6733) (-9.4561, -11.6692) (-9.4505, -11.6651) (-9.4449, -11.6609) (-9.4393, -11.6568) (-9.4338, -11.6527) (-9.4283, -11.6486) (-9.4228, -11.6446) (-9.4174, -11.6405) (-9.412, -11.6365) (-9.4067, -11.6324) (-9.4014, -11.6284) (-9.3962, -11.6244) (-9.3909, -11.6204) (-9.3858, -11.6164) (-9.3806, -11.6125) (-9.3755, -11.6085) (-9.3705, -11.6046) (-9.3654, -11.6007) (-9.3605, -11.5968) (-9.3555, -11.5929) (-9.3506, -11.589) (-9.3457, -11.5852) (-9.3409, -11.5813) (-9.3361, -11.5775) (-9.3314, -11.5737) (-9.3267, -11.5699) (-9.322, -11.5662) (-9.3174, -11.5624) (-9.3128, -11.5587) (-9.3083, -11.555) (-9.3038, -11.5513) (-9.2993, -11.5476) (-9.2949, -11.544) (-9.2905, -11.5403) (-9.2862, -11.5367) (-9.2819, -11.5331) (-9.2776, -11.5295) (-9.2734, -11.526) (-9.2692, -11.5224) (-9.2651, -11.5189) (-9.261, -11.5154) (-9.257, -11.512) (-9.253, -11.5085) (-9.249, -11.5051) (-9.2451, -11.5017) (-9.2412, -11.4983) (-9.2373, -11.495) (-9.2335, -11.4916) (-9.2298, -11.4883) (-9.2261, -11.485) (-9.2224, -11.4818) (-9.2188, -11.4785) (-9.2152, -11.4753) (-9.2116, -11.4721) (-9.2081, -11.469) (-9.2047, -11.4658) (-9.2013, -11.4627) (-9.1979, -11.4597) (-9.1946, -11.4566) (-9.1913, -11.4536) (-9.188, -11.4506) (-9.1848, -11.4476) (-9.1817, -11.4447) (-9.1786, -11.4418) (-9.1755, -11.4389) (-9.1725, -11.436) (-9.1695, -11.4332) (-9.1666, -11.4304) (-9.1637, -11.4276) (-9.1608, -11.4249) (-9.158, -11.4222) (-9.1553, -11.4195) (-9.1526, -11.4169) (-9.1499, -11.4143) (-9.1473, -11.4117) (-9.1447, -11.4092) (-9.1422, -11.4067) (-9.1397, -11.4042) (-9.1372, -11.4018) (-9.1348, -11.3994) (-9.1325, -11.397) (-9.1302, -11.3947) (-9.1279, -11.3924) (-9.1257, -11.3902) (-9.1235, -11.388) (-9.1214, -11.3858) (-9.1194, -11.3836) (-9.1173, -11.3815) (-9.1153, -11.3795) (-9.1134, -11.3775) (-9.1115, -11.3755) (-9.1097, -11.3735) (-9.1079, -11.3717) (-9.1062, -11.3698) (-9.1045, -11.368) (-9.1028, -11.3662) (-9.1012, -11.3645) (-9.0997, -11.3628) (-9.0982, -11.3612) (-9.0967, -11.3596) (-9.0953, -11.3581) (-9.0939, -11.3566) (-9.0926, -11.3551) (-9.0914, -11.3537) (-9.0902, -11.3524) (-9.089, -11.3511) (-9.0879, -11.3498) (-9.0868, -11.3486) (-9.0858, -11.3475) (-9.0849, -11.3464) (-9.084, -11.3453) (-9.0831, -11.3443) (-9.0823, -11.3434) (-9.0815, -11.3425) (-9.0808, -11.3417) (-9.0802, -11.3409) (-9.0796, -11.3402) (-9.079, -11.3395) (-9.0785, -11.3389) (-9.0781, -11.3384) (-9.0777, -11.3379) (-9.0773, -11.3375) (-9.0771, -11.3372) (-9.0769, -11.337) (-9.0769, -11.3369) (-9.0768, -11.3369) knots -1 -1 -1 -1 -1 -1 -0.99583333 -0.99166667 -0.9875 -0.98333333 -0.97916667 -0.975 -0.97083333 -0.96666667 -0.9625 -0.95833333 -0.95416667 -0.95 -0.94583333 -0.94166667 -0.9375 -0.93333333 -0.92916667 -0.925 -0.92083333 -0.91666667 -0.9125 -0.90833333 -0.90416667 -0.9 -0.89583333 -0.89166667 -0.8875 -0.88333333 -0.87916667 -0.875 -0.87083333 -0.86666667 -0.8625 -0.85833333 -0.85416667 -0.85 -0.84583333 -0.84166667 -0.8375 -0.83333333 -0.82916667 -0.825 -0.82083333 -0.81666667 -0.8125 -0.80833333 -0.80416667 -0.8 -0.79583333 -0.79166667 -0.7875 -0.78333333 -0.77916667 -0.775 -0.77083333 -0.76666667 -0.7625 -0.75833333 -0.75416667 -0.75 -0.74583333 -0.74166667 -0.7375 -0.73333333 -0.72916667 -0.725 -0.72083333 -0.71666667 -0.7125 -0.70833333 -0.70416667 -0.7 -0.69583333 -0.69166667 -0.6875 -0.68333333 -0.67916667 -0.675 -0.67083333 -0.66666667 -0.6625 -0.65833333 -0.65416667 -0.65 -0.64583333 -0.64166667 -0.6375 -0.63333333 -0.62916667 -0.625 -0.62083333 -0.61666667 -0.6125 -0.60833333 -0.60416667 -0.6 -0.59583333 -0.59166667 -0.5875 -0.58333333 -0.57916667 -0.575 -0.57083333 -0.56666667 -0.5625 -0.55833333 -0.55416667 -0.55 -0.54583333 -0.54166667 -0.5375 -0.53333333 -0.52916667 -0.525 -0.52083333 -0.51666667 -0.5125 -0.50833333 -0.50416667 -0.5 -0.49583333 -0.49166667 -0.4875 -0.48333333 -0.47916667 -0.475 -0.47083333 -0.46666667 -0.4625 -0.45833333 -0.45416667 -0.45 -0.44583333 -0.44166667 -0.4375 -0.43333333 -0.42916667 -0.425 -0.42083333 -0.41666667 -0.4125 -0.40833333 -0.40416667 -0.4 -0.39583333 -0.39166667 -0.3875 -0.38333333 -0.37916667 -0.375 -0.37083333 -0.36666667 -0.3625 -0.35833333 -0.35416667 -0.35 -0.34583333 -0.34166667 -0.3375 -0.33333333 -0.32916667 -0.325 -0.32083333 -0.31666667 -0.3125 -0.30833333 -0.30416667 -0.3 -0.29583333 -0.29166667 -0.2875 -0.28333333 -0.27916667 -0.275 -0.27083333 -0.26666667 -0.2625 -0.25833333 -0.25416667 -0.25 -0.24583333 -0.24166667 -0.2375 -0.23333333 -0.22916667 -0.225 -0.22083333 -0.21666667 -0.2125 -0.20833333 -0.20416667 -0.2 -0.19583333 -0.19166667 -0.1875 -0.18333333 -0.17916667 -0.175 -0.17083333 -0.16666667 -0.1625 -0.15833333 -0.15416667 -0.15 -0.14583333 -0.14166667 -0.1375 -0.13333333 -0.12916667 -0.125 -0.12083333 -0.11666667 -0.1125 -0.10833333 -0.10416667 -0.1 -0.09583333 -0.09166667 -0.0875 -0.08333333 -0.07916667 -0.075 -0.07083333 -0.06666667 -0.0625 -0.05833333 -0.05416667 -0.05 -0.04583333 -0.04166667 -0.0375 -0.03333333 -0.02916667 -0.025 -0.02083333 -0.01666667 -0.0125 -0.00833333 -0.00416667 0 0 0 0 0 0
  arc A53 (14.7969, 6.087) -> (14.4246, 6.9233) centre (0, 0) ccw
  line L86 (10.3255, 10.2117) -> (10.326, 10.2121)